# Autodesk Inventor part: LED
Saved by Autodesk Inventor 2013 (Build 170138000, 138)
## iProperties
Created: 2013-01-27
Part Number: LED
Material: Generic
Document SubType Name: Modeling
Designer: davidgitz
Density: 1 g/cm^3
Author: davidgitz
Autodesk Inventor part; units mm, degrees
ref_plane "YZ Plane" through (0, 0, 0) normal (1, 0, 0) x (0, 1, 0)
ref_plane "XZ Plane" through (0, 0, 0) normal (0, 1, 0) x (-1, 0, 0)
ref_plane "XY Plane" through (0, 0, 0) normal (0, 0, 1) x (1, 0, 0)
sketch "LEDT175, LED_28" plane through (0, 0, 0) normal (0, 0, 1) x (1, 0, 0)
  arc A0 (-2.794, -1.27) -> (0, -4.064) centre (0, -1.27) ccw
  arc A1 (0, -4.064) -> (2.794, -1.27) centre (0, -1.27) ccw
  arc A2 (2.794, -1.27) -> (1.7018, 1.3462) centre (-0.9101, -1.2803) ccw
  line L0 (1.7018, 1.3462) -> (-1.7018, 1.3462)
  arc A3 (-1.7018, 1.3462) -> (-2.794, -1.27) centre (0.9101, -1.2803) ccw
  constraints: 8 point on circle, 4 centre point, 2 end point
extrude "Extrusion1" add sketch "LEDT175, LED_28" along normal blind 3
body "Solid1"
